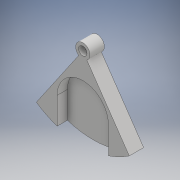
# Autodesk Inventor part: RescueKitThrow-Joint
Saved by Autodesk Inventor 2018.3 (Build 223284000, 284)
## iProperties
Created: 2019-02-13
Part Number: RescueKitThrow-Joint
Material: 一般
Document SubType Name: Modeling
Designer: TOMOKI
Density: 1 g/cm^3
Appearance: 既定
Author: TOMOKI
Autodesk Inventor part; units mm, degrees
ref_plane "YZ Plane" through (0, 0, 0) normal (1, 0, 0) x (0, 1, 0)
ref_plane "XZ Plane" through (0, 0, 0) normal (0, 1, 0) x (-1, 0, 0)
ref_plane "XY Plane" through (0, 0, 0) normal (0, 0, 1) x (1, 0, 0)
sketch "スケッチ1" plane through (0, 0, 0) normal (0, 1, 0) x (-1, 0, 0)
  circle A0 centre (55, 15) radius 12.5
  arc A1 (32.3675, 7.0186) -> (77.6325, 7.0186) centre (55, 40) ccw
  arc A2 (56.9803, 37.1141) -> (53.0197, 37.1141) centre (55, 40) ccw
  line L0 (53.0197, 37.1141) -> (32.3675, 7.0186)
  line L1 (77.6325, 7.0186) -> (56.9803, 37.1141)
  point P0 (0, 0)
  constraints: 4 end point, 4 point on circle, 3 centre point
extrude "押し出し1" add sketch "スケッチ1" along normal blind 7
sketch "スケッチ2" plane through (0, 7, 0) normal (0, 1, 0) x (1, 0, 0)
  circle A0 centre (-55, -15) radius 12.5 projected
  circle A1 centre (-55, -15) radius 12.5
  point P0 (0, 0)
  constraints: 1 centre point, 1 coincident
extrude "押し出し2" add sketch "スケッチ2" against normal blind 2
sketch "スケッチ3" plane through (0, 0, 0) normal (0, -1, 0) x (1, 0, 0)
  circle A0 centre (-55, 15) radius 12.5 projected
  line L0 (-67.5, 15) -> (-42.5, 15)
  line L1 (-42.5, 15) -> (-42.5, -1.7653)
  line L2 (-42.5, -1.7653) -> (-67.5, -1.7653)
  line L3 (-67.5, -1.7653) -> (-67.5, 15)
  point P0 (0, 0)
  constraints: 8 end point, 2 parallel, 1 horizontal, 1 horizontal alignment, 1 perpendicular, 1 other
extrude "押し出し3" cut sketch "スケッチ3" against normal blind 5 contours L1 L2 L3 A0 | A0 L0 picked at (-57.3669, 11.5709)
sketch "スケッチ4" plane through (0, 0, 0) normal (0, -1, 0) x (1, 0, 0)
  line L0 (-67.5, 2.0033) -> (-67.5, 15) projected
  arc A0 (-42.5, 15) -> (-67.5, 15) centre (-55, 15) ccw projected
  line L1 (-42.5, 15) -> (-42.5, 2.0033) projected
  arc A1 (-42.5, 2.0033) -> (-32.3675, 7.0186) centre (-55, 40) ccw projected
  line L2 (-32.3675, 7.0186) -> (-53.0197, 37.1141) projected
  arc A2 (-53.0197, 37.1141) -> (-56.9803, 37.1141) centre (-55, 40) ccw projected
  line L3 (-56.9803, 37.1141) -> (-77.6325, 7.0186) projected
  arc A3 (-77.6325, 7.0186) -> (-67.5, 2.0033) centre (-55, 40) ccw projected
  circle A4 centre (-55, 40) radius 2.05
  point P0 (0, 0)
  dimension "d12" = 4.1
  constraints: 1 centre point, 1 coincident
  measures "d12" diameter of A4
extrude "押し出し4" cut sketch "スケッチ4" against normal blind 2.8 contours A4
sketch "スケッチ5" plane through (0, 7, 0) normal (0, 1, 0) x (1, 0, 0)
  arc A0 (-32.3675, -7.0186) -> (-77.6325, -7.0186) centre (-55, -40) ccw projected
  line L0 (-77.6325, -7.0186) -> (-56.9803, -37.1141) projected
  arc A1 (-56.9803, -37.1141) -> (-53.0197, -37.1141) centre (-55, -40) ccw projected
  line L1 (-53.0197, -37.1141) -> (-32.3675, -7.0186) projected
  circle A2 centre (-55, -40) radius 1.25
  point P0 (0, 0)
  dimension "d15" = 2.5
  constraints: 1 centre point, 1 coincident
  measures "d15" diameter of A2
extrude "押し出し5" cut sketch "スケッチ5" against normal blind 5 contours A2
